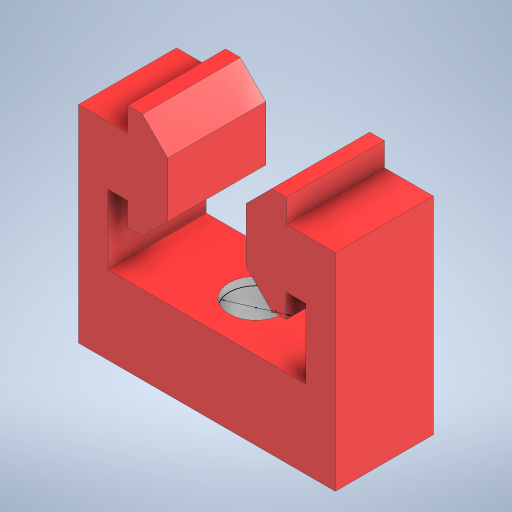
# Autodesk Inventor part: sostenedor_part1
Saved by Autodesk Inventor 2023.2 (Build 272271030, 271C)
## iProperties
Created: 2023-03-04
Part Number: sostenedor_part1
Material: Generic
Document SubType Name: Modeling
Designer: Cris Pat
Density: 1 g/cm^3
Appearance: Default
Author: Cris Pat
Autodesk Inventor part; units mm, degrees
ref_plane "YZ Plane" through (0, 0, 0) normal (1, 0, 0) x (0, 1, 0)
ref_plane "XY Plane" through (0, 0, 0) normal (0, 0, 1) x (1, 0, 0)
sketch "Sketch1" plane through (0, 0, 0) normal (0, 0, 1) x (1, 0, 0)
  line L0 (-10, 13.1) -> (10, 13.1) construction
  line L1 (10, 13.1) -> (10, -6.9) construction
  line L2 (10, -6.9) -> (-10, -6.9) construction
  line L3 (-10, -6.9) -> (-10, 13.1) construction
  line L4 (0, 13.1) -> (0, -6.9) construction
  circle A0 centre (0, 3.1) radius 2.5 construction
  line L5 (10, 3.1) -> (-10, 3.1) construction
  line L6 (0, 3.1) -> (10, 13.1) construction
  line L7 (-3.9, 7) -> (3.9, 7) construction
  line L8 (3.9, 7) -> (3.9, -0.8) construction
  line L9 (3.9, -0.8) -> (-3.9, -0.8) construction
  line L10 (-3.9, -0.8) -> (-3.9, 7) construction
  line L11 (2.8393, 7) -> (3.9, 5.9393) construction
  line L12 (10, 13.1) -> (5.5, 13.1) construction
  line L13 (5.5, 13.1) -> (5.5, 8.6) construction
  line L14 (5.5, 8.6) -> (10, 8.6) construction
  line L15 (10, 8.6) -> (10, 13.1) construction
  line L16 (3.9, 3.1) -> (3.9, 5.9393) construction
  line L17 (3.9, 5.9393) -> (6.5607, 8.6) construction
  line L18 (0, 7) -> (2.8393, 7) construction
  line L19 (2.8393, 7) -> (5.5, 9.6607) construction
  line L20 (10, 13.1) -> (10, 6.2) construction
  line L21 (10, 6.2) -> (8.2, 6.2) construction
  line L22 (8.2, 6.2) -> (8.2, 8.6) construction
  line L23 (6.5607, 8.6) -> (8.2, 8.6) construction
  line L24 (10, 13.1) -> (3.1, 13.1) construction
  line L25 (3.1, 13.1) -> (3.1, 11.3) construction
  line L26 (3.1, 11.3) -> (5.5, 11.3) construction
  line L27 (5.5, 9.6607) -> (5.5, 11.3) construction
  line L28 (-3.9, 3.1) -> (-3.9, 5.9393) construction
  line L29 (-3.9, 5.9393) -> (-6.5607, 8.6) construction
  line L30 (-6.5607, 8.6) -> (-8.2, 8.6) construction
  line L31 (-8.2, 6.2) -> (-8.2, 8.6) construction
  line L32 (-10, 6.2) -> (-8.2, 6.2) construction
  line L33 (-10, 13.1) -> (-10, 6.2) construction
  line L34 (-10, 13.1) -> (-3.1, 13.1) construction
  line L35 (-3.1, 13.1) -> (-3.1, 11.3) construction
  line L36 (-3.1, 11.3) -> (-5.5, 11.3) construction
  line L37 (-5.5, 9.6607) -> (-5.5, 11.3) construction
  line L38 (-2.8393, 7) -> (-5.5, 9.6607) construction
  line L39 (0, 7) -> (-2.8393, 7) construction
  line L40 (-3.9, 3.1) -> (-3.9, 0.2607) construction
  line L41 (-3.9, 0.2607) -> (-6.5607, -2.4) construction
  line L42 (-6.5607, -2.4) -> (-8.2, -2.4) construction
  line L43 (-8.2, 0) -> (-8.2, -2.4) construction
  line L44 (-10, 0) -> (-8.2, 0) construction
  line L45 (-10, -6.9) -> (-10, 0) construction
  line L46 (-10, -6.9) -> (-3.1, -6.9) construction
  line L47 (-3.1, -6.9) -> (-3.1, -5.1) construction
  line L48 (-3.1, -5.1) -> (-5.5, -5.1) construction
  line L49 (-5.5, -3.4607) -> (-5.5, -5.1) construction
  line L50 (-2.8393, -0.8) -> (-5.5, -3.4607) construction
  line L51 (0, -0.8) -> (-2.8393, -0.8) construction
  line L52 (0, -0.8) -> (2.8393, -0.8) construction
  line L53 (2.8393, -0.8) -> (5.5, -3.4607) construction
  line L54 (5.5, -3.4607) -> (5.5, -5.1) construction
  line L55 (3.1, -5.1) -> (5.5, -5.1) construction
  line L56 (3.1, -6.9) -> (3.1, -5.1) construction
  line L57 (10, -6.9) -> (3.1, -6.9) construction
  line L58 (10, -6.9) -> (10, 0) construction
  line L59 (10, 0) -> (8.2, 0) construction
  line L60 (8.2, 0) -> (8.2, -2.4) construction
  line L61 (6.5607, -2.4) -> (8.2, -2.4) construction
  line L62 (3.9, 0.2607) -> (6.5607, -2.4) construction
  line L63 (3.9, 3.1) -> (3.9, 0.2607) construction
  line L64 (-10.1, 0.1) -> (-8.1, 0.1)
  line L65 (-8.1, 0.1) -> (-8.1, -2.3)
  line L66 (-8.1, -2.3) -> (-6.6021, -2.3)
  line L67 (-6.6021, -2.3) -> (-4, 0.3021)
  line L68 (-4, 0.3021) -> (-4, 3.1)
  line L69 (-4, 3.1) -> (-4, 5.8979)
  line L70 (-4, 5.8979) -> (-6.6021, 8.5)
  line L71 (-6.6021, 8.5) -> (-8.1, 8.5)
  line L72 (-8.1, 8.5) -> (-8.1, 6.1)
  line L73 (-8.1, 6.1) -> (-10.5, 6.1)
  line L74 (-10.1, 0.1) -> (-10.1, -6.99)
  line L75 (-10.1, -6.99) -> (0, -6.99)
  line L76 (0, -6.9) -> (0, -6.99) construction
  line L77 (0.2, -14.99) -> (-13.1, -14.99)
  line L78 (-13.1, -14.99) -> (-13.1, 6.1)
  line L79 (-13.1, 6.1) -> (-10.5, 6.1)
  line L80 (10.1, 0.1) -> (8.1, 0.1)
  line L81 (8.1, 0.1) -> (8.1, -2.3)
  line L82 (8.1, -2.3) -> (6.6021, -2.3)
  line L83 (6.6021, -2.3) -> (4, 0.3021)
  line L84 (4, 0.3021) -> (4, 3.1)
  line L85 (4, 3.1) -> (4, 5.8979)
  line L86 (4, 5.8979) -> (6.6021, 8.5)
  line L87 (6.6021, 8.5) -> (8.1, 8.5)
  line L88 (8.1, 8.5) -> (8.1, 6.1)
  line L89 (8.1, 6.1) -> (10.5, 6.1)
  line L90 (10.1, 0.1) -> (10.1, -6.99)
  line L91 (10.1, -6.99) -> (0, -6.99)
  line L92 (0.2, -14.99) -> (13.1, -14.99)
  line L93 (13.1, -14.99) -> (13.1, 6.1)
  line L94 (13.1, 6.1) -> (10.5, 6.1)
  point P0 (0, 0)
  point P1 (9.1, 0)
  point P2 (-9.1, 0)
  point P3 (-5.2303, 7.2697)
  point P4 (-10, -3.45)
  point P5 (-5.05, -6.99)
  dimension "d0" = 20
  dimension "d1" = 20
  dimension "d2" = 5
  dimension "d3" = 6.1
  dimension "d4" = 6.1
  dimension "d5" = 1.5
  dimension "d6" = 4.5
  dimension "d7" = 4.5
  dimension "d8" = 1.5
  dimension "d9" = 6.9
  dimension "d10" = 1.8
  dimension "d13" = 3
  dimension "d14" = 0.1
  dimension "d17" = 0.1
  dimension "d18" = 0.09
  dimension "d31" = 8
  constraints: 190 end point, 49 symmetric about line, 13 midpoint, 9 perpendicular, 7 parallel, 6 point on line, 4 horizontal alignment, 3 horizontal, 3 vertical, 3 vertical alignment, 2 collinear, 1 centre point, 1 coincident, 9 other
  measures "d0" distance of L1.end L45.start
  measures "d1" distance of L6.end L1.end
  measures "d2" diameter of A0
  measures "d3" distance between parallel lines of L2 L9
  measures "d4" distance between parallel lines of L3 L10
  measures "d5" distance of L11.start L11.end
  measures "d6" distance between parallel lines of L1 L13
  measures "d7" distance between parallel lines of L0 L14
  measures "d8" distance between parallel lines of L17 L19
  measures "d9" distance of L6.end L21.start
  measures "d10" distance of L21.start L22.start
  measures "d13" distance between parallel lines of L78 L74
  measures "d14" distance from line of L64 point (-9.1, 0)
  measures "d17" distance from line of point (-10, -3.45) L74
  measures "d18" distance from line of point (-5.05, -6.99) L2
  measures "d31" distance between parallel lines of L77 L75
extrude "Extrusion1" add sketch "Sketch1" along normal mid plane 10
ref_plane "Work Plane1" through (0, -7.8, 0) normal (0, 1, 0) x (-1, 0, 0)
sketch "Sketch2" plane through (0, -7.8, 0) normal (0, 1, 0) x (-1, 0, 0)
  circle A0 centre (0, 0) radius 2.75
  dimension "d22" = 5.5
  constraints: 1 centre point, 1 coincident
  measures "d22" diameter of A0
extrude "Extrusion3" cut sketch "Sketch2" along normal through all both and the other way through all
body "Solid1"
